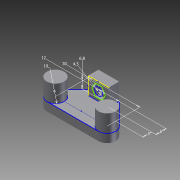
# Autodesk Inventor part: X_Belt
Saved by Autodesk Inventor 2012 (Build 160160000, 160)
## iProperties
Created: 2012-07-05
Part Number: X_Belt
Material: Default
Document SubType Name: Modeling
Designer: Administrator
Density: 1 g/cm^3
Author: Administrator
Autodesk Inventor part; units mm, degrees
ref_plane "YZ Plane" through (0, 0, 0) normal (1, 0, 0) x (0, 1, 0)
ref_plane "XZ Plane" through (0, 0, 0) normal (0, 1, 0) x (-1, 0, 0)
ref_plane "XY Plane" through (0, 0, 0) normal (0, 0, 1) x (1, 0, 0)
sketch "Sketch1" plane through (0, 0, 0) normal (0, 0, 1) x (1, 0, 0)
  circle A0 centre (15, 0) radius 5
  circle A1 centre (-15, 0) radius 5
  line L0 (-15, 0) -> (15, 0) construction
  line L1 (-6, 16) -> (6, 16)
  line L2 (6, 16) -> (6, 10)
  line L3 (6, 10) -> (-6, 10)
  line L4 (-6, 10) -> (-6, 16)
  line L5 (-6, 16) -> (-18.5255, 3.5456)
  line L6 (6, 16) -> (18.5255, 3.5456)
  line L7 (-15, -5) -> (15, -5)
  point P0 (0, 0)
  point P1 (0, 0)
  point P2 (0, 10)
  dimension "d0" = 10
  dimension "d1" = 12
  dimension "d2" = 6
  dimension "d3" = 30
  dimension "d5" = 5
  constraints: 16 end point, 4 point on circle, 3 tangent, 2 centre point, 2 horizontal, 2 midpoint, 2 parallel, 2 perpendicular, 1 coincident, 1 equal radius, 1 vertical alignment
  measures "d0" diameter of A1
  measures "d1" distance of L1.start L1.end
  measures "d2" distance of L1.end L2.end
  measures "d3" distance of L0.end L0.start
  measures "d5" distance edge to line of A0 L3
extrude "Extrusion1" add sketch "Sketch1" against normal blind 5
extrude "Extrusion2" add sketch "Sketch1" along normal blind 10 contours A0 | L2 L3 L4 L1 | A1
sketch "Sketch2" plane through (-6, 10, 10) normal (0, -1, 0) x (1, 0, 0)
  line L0 (12, 0) -> (0, 0) projected
  line L1 (0, -10) -> (0, 0) projected
  line L2 (9.926, -5) -> (7.963, -8.4)
  line L3 (7.963, -8.4) -> (4.037, -8.4)
  line L4 (4.037, -8.4) -> (2.074, -5)
  line L5 (2.074, -5) -> (4.037, -1.6)
  line L6 (4.037, -1.6) -> (7.963, -1.6)
  line L7 (7.963, -1.6) -> (9.926, -5)
  circle A0 centre (6, -5) radius 2.25
  point P0 (6, -10)
  point P1 (0, -5)
  point P2 (6, 0)
  dimension "d10" = 6.8
  dimension "d11" = 4.5
  constraints: 12 end point, 2 midpoint, 1 centre point, 1 coincident, 1 horizontal alignment, 1 vertical alignment, 13 other
  measures "d10" distance between parallel lines of L3 L6
  measures "d11" diameter of A0
extrude "Extrusion3" cut sketch "Sketch2" against normal blind 2 contours L2 L3 L4 L5 L6 L7 | A0
extrude "Extrusion4" cut sketch "Sketch2" against normal through all contours A0
body "Solid1"
